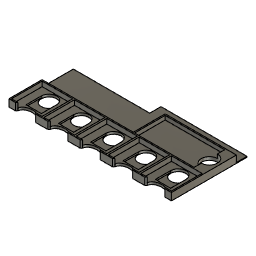
Food_Chain_Magnate_Garden_Restaurants v1 (Autodesk Fusion 360 design; units mm, degrees)
Autodesk Fusion 360 part; units mm, degrees
sketch "Sketch1" plane through (0, 0, 0) normal (0, 0, 1) x (1, 0, 0)
  line L0 (-75, 50) -> (20, 50)
  line L1 (127, 50) -> (127, -30)
  line L2 (-75, -30) -> (-75, 50)
  line L3 (20, 50) -> (20, 64)
  line L4 (127, 50) -> (127, 64)
  line L5 (127, 64) -> (20, 64)
  line L6 (-73.4, -28.4) -> (-73.4, 9.6)
  line L7 (-35.4, 9.6) -> (-35.4, -28.4)
  line L8 (-73.4, 9.6) -> (-35.4, -28.4) construction
  line L9 (-73.4, -28.4) -> (-35.4, 9.6) construction
  line L10 (-54.4, -9.4) -> (-54.4, -10.4)
  line L11 (-44.9, -0.9) -> (-63.9, -0.9)
  line L12 (-63.9, -0.9) -> (-63.9, -19.9)
  line L13 (-63.9, -19.9) -> (-44.9, -19.9)
  line L14 (-44.9, -19.9) -> (-44.9, -0.9)
  line L15 (-44.9, -0.9) -> (-63.9, -19.9) construction
  line L16 (-63.9, -0.9) -> (-44.9, -19.9) construction
  circle A0 centre (-54.4, -0.9) radius 9.5
  line L17 (-65.4, -28.4) -> (-65.4, -28.5)
  line L18 (-43.4, -28.4) -> (-43.4, -28.5)
  ellipse E0 centre (-54.4007, -28.4) end of major axis (-65.4, -28.4) minor radius 7 (-43.4014, -28.4001) -> (-65.4, -28.4) ccw
  line L19 (-66.9, -30) -> (-75, -30)
  line L20 (-43.4014, -28.4001) -> (-43.4, -28.4) construction
  line L21 (-65.4, -28.5) -> (-66.9, -30)
  line L22 (-43.4, -28.5) -> (-41.9, -30)
  line L23 (-65.4, -28.5) -> (-66.9, -30)
  line L24 (-44.9, -19.9) -> (-44.9, -0.9)
  line L25 (-43.4014, -28.4001) -> (-43.4, -28.4) construction
  line L26 (-73.4, -28.4) -> (-73.4, 9.6)
  circle A1 centre (-54.4, -0.9) radius 9.5
  line L27 (-73.4, -28.4) -> (-35.4, 9.6) construction
  line L28 (-43.4, -28.4) -> (-43.4, -28.5)
  line L29 (-35.4, 9.6) -> (-35.4, -28.4)
  line L30 (-73.4, 9.6) -> (-35.4, -28.4) construction
  line L31 (-54.4, -9.4) -> (-54.4, -10.4)
  line L32 (-63.9, -0.9) -> (-63.9, -19.9)
  line L33 (-44.9, -0.9) -> (-63.9, -19.9) construction
  line L34 (-44.9, -0.9) -> (-63.9, -0.9)
  line L35 (-63.9, -0.9) -> (-44.9, -19.9) construction
  line L36 (-65.4, -28.4) -> (-65.4, -28.5)
  line L37 (-43.4, -28.5) -> (-41.9, -30)
  ellipse E1 centre (-54.4007, -28.4) end of major axis (-65.4, -28.4) minor radius 7 (-43.4014, -28.4001) -> (-65.4, -28.4) ccw
  line L38 (-63.9, -19.9) -> (-44.9, -19.9)
  line L39 (-33.2, 9.6) -> (-33.2, -28.4)
  line L40 (4.8, 9.6) -> (4.8, -28.4)
  line L41 (7, 9.6) -> (7, -28.4)
  line L42 (45, 9.6) -> (45, -28.4)
  line L43 (47.2, 9.6) -> (47.2, -28.4)
  line L44 (85.2, 9.6) -> (85.2, -28.4)
  line L45 (87.4, 9.6) -> (87.4, -28.4)
  line L46 (125.4, 9.6) -> (125.4, -28.4)
  line L47 (-33.2, 9.6) -> (4.8, -28.4) construction
  line L48 (-33.2, -28.4) -> (4.8, 9.6) construction
  line L49 (7, 9.6) -> (45, -28.4) construction
  line L50 (7, -28.4) -> (45, 9.6) construction
  line L51 (47.2, 9.6) -> (85.2, -28.4) construction
  line L52 (47.2, -28.4) -> (85.2, 9.6) construction
  line L53 (87.4, 9.6) -> (125.4, -28.4) construction
  line L54 (87.4, -28.4) -> (125.4, 9.6) construction
  line L55 (-14.2, -9.4) -> (-14.2, -10.4) construction
  line L56 (26, -9.4) -> (26, -10.4) construction
  line L57 (66.2, -9.4) -> (66.2, -10.4) construction
  line L58 (106.4, -9.4) -> (106.4, -10.4) construction
  line L59 (-23.7, -0.9) -> (-4.7, -0.9)
  line L60 (-4.7, -0.9) -> (-4.7, -19.9)
  line L61 (-4.7, -19.9) -> (-23.7, -19.9)
  line L62 (-23.7, -19.9) -> (-23.7, -0.9)
  line L63 (-23.7, -0.9) -> (-4.7, -19.9) construction
  line L64 (-4.7, -0.9) -> (-23.7, -19.9) construction
  line L65 (16.5, -19.9) -> (35.5, -19.9)
  line L66 (35.5, -19.9) -> (35.5, -0.9)
  line L67 (35.5, -0.9) -> (16.5, -0.9)
  line L68 (16.5, -0.9) -> (16.5, -19.9)
  line L69 (16.5, -19.9) -> (35.5, -0.9) construction
  line L70 (35.5, -19.9) -> (16.5, -0.9) construction
  line L71 (75.7, -19.9) -> (56.7, -19.9)
  line L72 (56.7, -19.9) -> (56.7, -0.9)
  line L73 (56.7, -0.9) -> (75.7, -0.9)
  line L74 (75.7, -0.9) -> (75.7, -19.9)
  line L75 (75.7, -19.9) -> (56.7, -0.9) construction
  line L76 (56.7, -19.9) -> (75.7, -0.9) construction
  line L77 (115.9, -0.9) -> (96.9, -0.9)
  line L78 (96.9, -0.9) -> (96.9, -19.9)
  line L79 (96.9, -19.9) -> (115.9, -19.9)
  line L80 (115.9, -19.9) -> (115.9, -0.9)
  line L81 (115.9, -0.9) -> (96.9, -19.9) construction
  line L82 (96.9, -0.9) -> (115.9, -19.9) construction
  circle A2 centre (-14.2, -0.9) radius 9.5
  circle A3 centre (26, -0.9) radius 9.5
  circle A4 centre (66.2, -0.9) radius 9.5
  circle A5 centre (106.4, -0.9) radius 9.5
  line L83 (-25.2, -28.4) -> (-25.2, -28.5)
  line L84 (-3.2, -28.4) -> (-3.2, -28.5)
  line L85 (15, -28.4) -> (15, -28.5)
  line L86 (37, -28.4) -> (37, -28.5)
  line L87 (55.2, -28.4) -> (55.2, -28.5)
  line L88 (77.2, -28.4) -> (77.2, -28.5)
  line L89 (95.4, -28.4) -> (95.4, -28.5)
  line L90 (117.4, -28.4) -> (117.4, -28.5)
  line L91 (127, -30) -> (118.9, -30)
  ellipse E2 centre (106.4, -28.4) end of major axis (95.4, -28.4) minor radius 7 (117.4, -28.4) -> (95.4, -28.4) ccw
  ellipse E3 centre (66.2, -28.4) end of major axis (55.2, -28.4) minor radius 7 (77.2, -28.4) -> (55.2, -28.4) ccw
  line L92 (93.9, -30) -> (78.7, -30)
  line L93 (53.7, -30) -> (38.5, -30)
  ellipse E4 centre (-14.2, -28.4) end of major axis (-25.2, -28.4) minor radius 7 (-3.2, -28.4158) -> (-25.2, -28.4) ccw
  line L94 (13.5, -30) -> (-1.7, -30)
  line L95 (-26.7, -30) -> (-41.9, -30)
  line L96 (-3.2, -28.4158) -> (-3.2, -28.4158) construction
  ellipse E5 centre (26, -28.4) end of major axis (15, -28.4) minor radius 7 (37, -28.4) -> (15, -28.4) ccw
  line L97 (-26.7, -30) -> (-25.2, -28.5)
  line L98 (-3.2, -28.5) -> (-1.7, -30)
  line L99 (13.5, -30) -> (15, -28.5)
  line L100 (37, -28.5) -> (38.5, -30)
  line L101 (55.2, -28.5) -> (53.7, -30)
  line L102 (77.2, -28.5) -> (78.7, -30)
  line L103 (95.4, -28.5) -> (93.9, -30)
  line L104 (117.4, -28.5) -> (118.9, -30)
  line L105 (114, 11.2) -> (114, 49.2)
  line L106 (114, 49.2) -> (40, 49.2)
  line L107 (40, 49.2) -> (40, 11.2)
  circle A6 centre (114, 30.2) radius 10
  line L108 (115.6, 50.8) -> (38.4, 50.8)
  line L109 (38.4, 50.8) -> (38.4, 11.2)
  line L110 (115.6, 50.8) -> (127, 50.8)
  line L111 (87.4, 9.6) -> (125.4, 9.6)
  line L112 (-75, 11.2) -> (38.4, 11.2)
  line L113 (40, 11.2) -> (114, 11.2)
  line L114 (47.2, 9.6) -> (85.2, 9.6)
  line L115 (87.4, -28.4) -> (125.4, -28.4)
  line L116 (47.2, -28.4) -> (85.2, -28.4)
  line L117 (7, 9.6) -> (45, 9.6)
  line L118 (7, -28.4) -> (45, -28.4)
  line L119 (-73.4, -28.4) -> (-35.4, -28.4)
  line L120 (-33.2, -28.4) -> (4.8, -28.4)
  line L121 (-73.4, 9.6) -> (-35.4, 9.6)
  line L122 (-33.2, 9.6) -> (4.8, 9.6)
  point P0 (-54.4, -10.4)
  point P1 (-65.4, -30)
  point P2 (-43.4, -30)
  point P3 (-43.4, -30)
  point P4 (-65.4, -30)
  point P5 (-54.4, -10.4)
  point P6 (-14.2, -10.4)
  point P7 (26, -10.4)
  point P8 (66.2, -10.4)
  point P9 (106.4, -10.4)
  point P10 (-25.2, -30)
  point P11 (-3.2, -30)
  point P12 (15, -30)
  point P13 (37, -30)
  point P14 (55.2, -30)
  point P15 (77.2, -30)
  point P16 (95.4, -30)
  point P17 (117.4, -30)
  dimension "d1" = 202
  dimension "d2" = 80
  dimension "d3" = 14
  dimension "d4" = 95
  dimension "d5" = 1.6
  dimension "d6" = 38
  dimension "d7" = 1.6
  dimension "d8" = 1.6
  dimension "d9" = 38
  dimension "d11" = 1
  dimension "d12" = 19
  dimension "d13" = 19
  dimension "d14" = 19
  dimension "d15" = 8
  dimension "d16" = 8
  dimension "d18" = 1.5
  dimension "d19" = 1.5
  dimension "d20" = 1.5
  dimension "d21" = 1.5
  dimension "d22" = 38
  dimension "d23" = 1
  dimension "d24" = 19
  dimension "d25" = 19
  dimension "d26" = 19
  dimension "d27" = 8
  dimension "d28" = 8
  dimension "d29" = 1.5
  dimension "d30" = 1.5
  dimension "d31" = 1.5
  dimension "d32" = 1.5
  dimension "d33" = 2.2
  dimension "d34" = 38
  dimension "d35" = 2.2
  dimension "d36" = 38
  dimension "d37" = 2.2
  dimension "d38" = 38
  dimension "d39" = 2.2
  dimension "d40" = 38
  dimension "d41" = 1
  dimension "d42" = 1
  dimension "d43" = 1
  dimension "d44" = 1
  dimension "d45" = 19
  dimension "d46" = 19
  dimension "d47" = 19
  dimension "d48" = 19
  dimension "d49" = 19
  dimension "d50" = 19
  dimension "d51" = 19
  dimension "d52" = 19
  dimension "d53" = 19
  dimension "d54" = 19
  dimension "d55" = 19
  dimension "d56" = 19
  dimension "d57" = 8
  dimension "d58" = 8
  dimension "d59" = 8
  dimension "d60" = 8
  dimension "d61" = 8
  dimension "d62" = 8
  dimension "d63" = 8
  dimension "d64" = 8
  dimension "d65" = 14
  dimension "d66" = 14
  dimension "d67" = 14
  dimension "d68" = 14
  dimension "d69" = 1.5
  dimension "d70" = 1.5
  dimension "d71" = 1.5
  dimension "d72" = 1.5
  dimension "d73" = 1.5
  dimension "d74" = 1.5
  dimension "d75" = 1.5
  dimension "d76" = 1.5
  dimension "d77" = 1.5
  dimension "d78" = 1.5
  dimension "d79" = 1.5
  dimension "d80" = 1.5
  dimension "d81" = 1.5
  dimension "d82" = 1.5
  dimension "d83" = 1.5
  dimension "d84" = 1.5
  dimension "d85" = 38
  dimension "d86" = 13
  dimension "d87" = 74
  dimension "d88" = 20
  constraint horizontal L0
  constraint vertical L1
  constraint horizontal L91
  constraint vertical L2
  constraint perpendicular L0 L3
  constraint perpendicular L0 L4
  constraint perpendicular L3 L5
  constraint perpendicular L1 L119
  constraint perpendicular L1 L121
  constraint coincident L2 L112.start
  constraint perpendicular L1 L112
  constraint perpendicular L6 L121
  constraint perpendicular L7 L119
  constraint midpoint L9 L10.start
  constraint vertical L10
  constraint horizontal L11
  constraint perpendicular L11 L12
  constraint parallel L11 L13
  constraint parallel L12 L14
  constraint coincident L15 P5
  constraint coincident L16 P5
  constraint coincident P5 P0
  constraint midpoint L11 A0.centre
  constraint coincident L17.start L119
  constraint coincident P4 L91
  constraint perpendicular L17 L91
  constraint coincident L18.start L119
  constraint perpendicular L18 L91
  constraint collinear L19 L91
  constraint coincident P4 L17
  constraint coincident P4 L19
  constraint coincident P3 L18
  constraint coincident P3 L91
  constraint midpoint L10.start L27
  constraint vertical L31
  constraint horizontal L34
  constraint perpendicular L32 L34
  constraint parallel L34 L38
  constraint parallel L24 L32
  constraint coincident P5 L33
  constraint coincident P5 L35
  constraint midpoint A0.centre L34
  constraint coincident P4 L36
  constraint coincident P3 L28
  constraint coincident L39.start L121
  constraint coincident L39.end L119
  constraint perpendicular L39 L119
  constraint perpendicular L40 L119
  constraint coincident L41.start L121
  constraint coincident L41.end L119
  constraint perpendicular L41 L119
  constraint perpendicular L42 L119
  constraint coincident L43.start L121
  constraint coincident L43.end L119
  constraint perpendicular L43 L119
  constraint perpendicular L44 L119
  constraint coincident L45.start L121
  constraint coincident L45.end L119
  constraint perpendicular L45 L121
  constraint coincident L46.end L119
  constraint perpendicular L46 L119
  constraint midpoint L48 L55.start
  constraint vertical L55
  constraint midpoint L50 L56.start
  constraint vertical L56
  constraint midpoint L52 L57.start
  constraint vertical L57
  constraint midpoint L53 L58.start
  constraint vertical L58
  constraint horizontal L59
  constraint perpendicular L59 L60
  constraint parallel L59 L61
  constraint parallel L60 L62
  constraint coincident L63 P6
  constraint coincident L64 P6
  constraint coincident P6 L55.end
  constraint horizontal L65
  constraint perpendicular L65 L66
  constraint parallel L65 L67
  constraint parallel L66 L68
  constraint coincident L69 P7
  constraint coincident L70 P7
  constraint coincident P7 L56.end
  constraint horizontal L71
  constraint perpendicular L71 L72
  constraint parallel L71 L73
  constraint parallel L72 L74
  constraint coincident L75 P8
  constraint coincident L76 P8
  constraint coincident P8 L57.end
  constraint horizontal L77
  constraint perpendicular L77 L78
  constraint parallel L77 L79
  constraint parallel L78 L80
  constraint coincident L81 P9
  constraint coincident L82 P9
  constraint coincident P9 L58.end
  constraint midpoint L59 A2.centre
  constraint midpoint L67 A3.centre
  constraint midpoint L73 A4.centre
  constraint midpoint L77 A5.centre
  constraint coincident L83.start L119
  constraint coincident P10 L91
  constraint perpendicular L83 L91
  constraint coincident L84.start L119
  constraint coincident P11 L91
  constraint perpendicular L84 L91
  constraint coincident L85.start L119
  constraint coincident P12 L91
  constraint perpendicular L85 L91
  constraint coincident L86.start L119
  constraint coincident P13 L91
  constraint perpendicular L86 L119
  constraint coincident L87.start L119
  constraint coincident P14 L91
  constraint perpendicular L87 L91
  constraint coincident L88.start L119
  constraint coincident P15 L91
  constraint perpendicular L88 L91
  constraint coincident L89.start L119
  constraint coincident P16 L91
  constraint perpendicular L89 L91
  constraint coincident L90.start L119
  constraint perpendicular L90 L91
  constraint coincident L84.start E4
  constraint collinear L91 L92
  constraint collinear L92 L93
  constraint collinear L93 L94
  constraint collinear L94 L95
  constraint coincident L84 L96.start
  constraint coincident P10 L83
  constraint coincident P11 L84
  constraint coincident P12 L85
  constraint coincident P13 L86
  constraint coincident P14 L87
  constraint coincident P15 L88
  constraint coincident P16 L89
  constraint coincident P16 L92
  constraint coincident P17 L90
  constraint coincident P17 L91
  constraint perpendicular L105 L112
  constraint perpendicular L105 L106
  constraint coincident L107.end L112
  constraint perpendicular L107 L112
  constraint midpoint L105 A6.centre
  constraint parallel L106 L108
  constraint parallel L107 L109
  constraint coincident L4 L110.end
  constraint perpendicular L4 L110
  constraint collinear L111 L121
  constraint collinear L112 L113
  constraint collinear L114 L121
  constraint collinear L115 L119
  constraint collinear L116 L119
  constraint collinear L117 L121
  constraint collinear L118 L119
  constraint collinear L119 L120
  constraint collinear L121 L122
  measures "d1" distance of L0.start L1.start
  measures "d2" distance of L0.start L2.start
  measures "d3" distance of L0.end L3.end
  measures "d4" distance of L2 L3
  measures "d5" distance of L91 L119
  measures "d6" distance of L119 L121
  measures "d7" distance of L112 L121
  measures "d8" distance of L2 L6
  measures "d9" distance of L6 L7
  measures "d11" distance of L10.start P5
  measures "d12" distance of L12.end L13.end
  measures "d13" distance of L11.end L12.end
  measures "d14" diameter of A0
  measures "d15" distance of L6 L17
  measures "d16" distance of L7 L18
  measures "d18" distance of P4 L17.end
  measures "d19" distance of P4 L19.start
  measures "d20" distance of P3 L18.end
  measures "d21" distance of P3 L22.end
  measures "d22" distance of L26 L29
  measures "d23" distance of L10.start P5
  measures "d24" distance of L12.end L13.end
  measures "d25" distance of L12.end L11.end
  measures "d26" diameter of A1
  measures "d27" distance of L26 L36
  measures "d28" distance of L28 L29
  measures "d29" distance of L17.end P4
  measures "d30" distance of L19.start P4
  measures "d31" distance of P3 L18.end
  measures "d32" distance of P3 L22.end
  measures "d33" distance of L7 L39
  measures "d34" distance of L39 L40
  measures "d35" distance of L40 L41
  measures "d36" distance of L41 L42
  measures "d37" distance of L42 L43
  measures "d38" distance of L43 L44
  measures "d39" distance of L44 L45
  measures "d40" distance of L45 L46
  measures "d41" distance of L55.start P6
  measures "d42" distance of L56.start P7
  measures "d43" distance of L57.start P8
  measures "d44" distance of L58.start P9
  measures "d45" distance of L60.end L61.end
  measures "d46" distance of L59.end L60.end
  measures "d47" distance of L66.end L67.end
  measures "d48" distance of L65.end L66.end
  measures "d49" distance of L72.end L73.end
  measures "d50" distance of L71.end L72.end
  measures "d51" distance of L78.end L79.end
  measures "d52" distance of L77.end L78.end
  measures "d53" diameter of A2
  measures "d54" diameter of A3
  measures "d55" diameter of A4
  measures "d56" diameter of A5
  measures "d57" distance of L39 L83
  measures "d58" distance of L40 L84
  measures "d59" distance of L46 L90
  measures "d60" distance of L45 L89
  measures "d61" distance of L44 L88
  measures "d62" distance of L43 L87
  measures "d63" distance of L42 L86
  measures "d64" distance of L41 L85
  measures "d69" distance of P10 L95.start
  measures "d70" distance of P10 L83.end
  measures "d71" distance of P11 L84.end
  measures "d72" distance of P11 L94.end
  measures "d73" distance of P12 L94.start
  measures "d74" distance of P12 L85.end
  measures "d75" distance of P13 L86.end
  measures "d76" distance of P13 L93.end
  measures "d77" distance of P14 L87.end
  measures "d78" distance of P14 L93.start
  measures "d79" distance of P15 L88.end
  measures "d80" distance of P15 L92.end
  measures "d81" distance of P16 L89.end
  measures "d82" distance of P16 L92.start
  measures "d83" distance of P17 L90.end
  measures "d84" distance of P17 L91.end
  measures "d85" distance of L105.start L105.end
  measures "d86" distance of L1 L105
  measures "d87" distance of L105.end L106.end
  measures "d88" diameter of A6
extrude "Extrude1" add sketch "Sketch1" along normal blind 4 contours L105 L106 L107 A6 L113 makes body 1
extrude "Extrude2" add sketch "Sketch1" along normal blind 1 separate body contours L12 L13 L14 A0 L24 A1 L32 L38 | L60 L61 L62 A2 | L65 L66 L68 A3 | L71 L72 L74 A4 | L78 L79 L80 A5 makes body 2 at (26.2366, -16.7245, 0) makes body 3 at (-13.9634, -16.7245, 0) makes body 4 at (66.4366, -16.7245, 0) makes body 5 at (-54.6366, -16.7245, 0) makes body 6 at (106.6366, -16.7245, 0)
extrude "Extrude3" add sketch "Sketch1" along normal blind 3 contours L6 L7 E0 L26 L29 E1 L119 L121 | L45 L46 E2 L111 L115 | L39 L40 E4 L120 L122 | L43 L44 E3 L114 L116 | L41 L42 E5 L117 L118 bodies 2 3 4 5 6
extrude "Extrude4" add sketch "Sketch1" along normal blind 9 contours L1 L2 L4 L6 L7 L17 L18 L19 L21 L22 L23 L26 L28 L29 L36 L37 L39 L40 L41 L42 L43 L44 L45 L46 L83 L84 L85 L86 L87 L88 L89 L90 L91 L92 L93 E4 L94 L95 L97 L98 L99 L100 L101 L102 L103 L104 L108 L109 L110 L111 L112 L114 L115 L116 L117 L118 L119 L120 L121 L122 bodies 1 2 3 4 5 6
extrude "Extrude5" add sketch "Sketch1" along normal blind 1 contours L0 L2 L3 L4 L5 L108 L109 L110 L112 bodies 1
equation "d19 = d18"
equation "d21 = d20"
equation "d30 = d18"
equation "d32 = d20"
equation "d70 = d69"
equation "d72 = d71"
equation "d74 = d73"
equation "d76 = d75"
equation "d78 = d77"
equation "d80 = d79"
equation "d82 = d81"
equation "d84 = d83"
